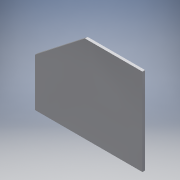
# Autodesk Inventor part: side plate
Saved by Autodesk Inventor 2016 (Build 200138000, 138)
## iProperties
Created: 2015-02-06
Part Number: side plate
Material: Aluminum 6061
Document SubType Name: Modeling
Designer: degan
Density: 2.7 g/cm^3
Appearance: Aluminum - Flat
Mass: 97.9398 g
Surface Area: 241.974 cm^2
Volume: 36.274 cm^3
Author: degan
Autodesk Inventor part; units mm, degrees
ref_plane "YZ Plane" through (0, 0, 0) normal (1, 0, 0) x (0, 1, 0)
ref_plane "XZ Plane" through (0, 0, 0) normal (0, 1, 0) x (-1, 0, 0)
ref_plane "XY Plane" through (0, 0, 0) normal (0, 0, 1) x (1, 0, 0)
sketch "Sketch2" plane through (0, 0, 0) normal (0, 0, 1) x (1, 0, 0)
  line L0 (0, 0) -> (0, -55.88)
  line L1 (0, 0) -> (55.88, 0) construction
  line L2 (0, -55.88) -> (125.6284, -55.88)
  line L3 (125.6284, -55.88) -> (125.6284, 45.72)
  line L4 (125.6284, 45.72) -> (58.5724, 45.72)
  line L5 (58.5724, 45.72) -> (0, 0)
  dimension "d4" = 55.88
  dimension "d5" = 90
  dimension "d6" = 125.6284
  dimension "d7" = 101.6
  dimension "d8" = 90
  dimension "d9" = 67.056
  dimension "d10" = 90
  constraints: 12 end point, 4 perpendicular, 1 horizontal, 1 vertical
  measures "d4" distance of L0.start L0.end
  measures "d5" angle of L0 L1
  measures "d6" distance of L0.end L2.end
  measures "d7" distance of L2.end L3.end
  measures "d8" angle of L3 L2
  measures "d9" distance of L3.end L4.end
  measures "d10" angle of L4 L3
extrude "Extrusion2" add sketch "Sketch2" along normal blind 3.175
body "Solid2"
